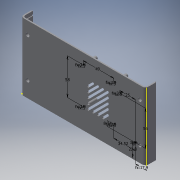
# Autodesk Inventor part: case-bottom
Saved by Autodesk Inventor 2017 (Build 210142000, 142)
## iProperties
Created: 2020-10-01
Part Number: case-bottom
Material: Generic
Document SubType Name: Modeling
Designer: jferner
Density: 1 g/cm^3
Appearance: Default
caseBottomDepth: 108.000 mm
caseBottomHeight: 17.000 mm
caseBottomWidth: 200.000 mm
thickness: 2.000 mm
fillet: 5.000 mm
frontBackOffset: -5.000 mm
filletInner: 3.000 mm
filletMid: 4.000 mm
lipHeight: 1.000 mm
offsetFromSideOfCase: 20.000 mm
caseJoinSpacingFrontBack: 63.000 mm
caseJoinSpacingLeftRight: 180.000 mm
caseJoinOffsetFromSide: 9.000 mm
caseJoinOffsetFromBack: 25.000 mm
caseJoinDiameter: 8.000 mm
holeDiameter: 3.400 mm
Author: jferner
Autodesk Inventor part; units mm, degrees
ref_plane "YZ Plane" through (0, 0, 0) normal (1, 0, 0) x (0, 1, 0)
ref_plane "XZ Plane" through (0, 0, 0) normal (0, 1, 0) x (-1, 0, 0)
ref_plane "XY Plane" through (0, 0, 0) normal (0, 0, 1) x (1, 0, 0)
sketch "Sketch1" plane through (0, 0, 0) normal (0, 0, 1) x (1, 0, 0)
  line L0 (0, 17) -> (0, 5)
  line L1 (5, 0) -> (195, 0)
  line L2 (200, 5) -> (200, 17)
  arc A0 (0, 5) -> (5, 0) centre (5, 5) ccw
  arc A1 (195, 0) -> (200, 5) centre (195, 5) ccw
  line L3 (2, 17) -> (2, 5)
  arc A2 (2, 5) -> (5, 2) centre (5, 5) ccw
  line L4 (5, 2) -> (195, 2)
  arc A3 (195, 2) -> (198, 5) centre (195, 5) ccw
  line L5 (198, 5) -> (198, 17)
  line L6 (0, 17) -> (2, 17)
  line L7 (198, 17) -> (200, 17)
  point P0 (0, 0)
  dimension "fillet" = 5
  dimension "thickness" = 2
  dimension "caseBottomWidth" = 200
  dimension "caseBottomHeight" = 17
  constraints: 16 end point, 8 point on circle, 4 centre point, 4 perpendicular, 4 tangent, 2 collinear, 2 point on line, 1 equal radius, 1 horizontal, 1 vertical, 4 other
  measures "fillet" radius of A0
  measures "thickness" distance between parallel lines of L0 L3
  measures "caseBottomWidth" distance between parallel lines of L2 L0
  measures "caseBottomHeight" distance between parallel lines of L6 L1
extrude "Extrusion1" add sketch "Sketch1" along normal blind 108
ref_plane "Work Plane1" through (0, 0, 103) normal (0, 0, 1) x (1, 0, 0)
sketch "Sketch3" plane through (0, 0, 103) normal (0, 0, 1) x (1, 0, 0)
  line L0 (2, 17) -> (1, 17)
  line L1 (2, 17) -> (2, 5)
  line L2 (1, 17) -> (1, 5)
  line L3 (195, 2) -> (5, 2) projected
  line L4 (195, 2) -> (5, 2)
  line L5 (198, 17) -> (198, 5) projected
  line L6 (198, 17) -> (198, 5)
  line L7 (198, 17) -> (199, 17)
  line L8 (199, 17) -> (199, 5)
  line L9 (5, 1) -> (195, 1)
  arc A0 (2, 5) -> (5, 2) centre (5, 5) ccw
  arc A1 (195, 2) -> (198, 5) centre (195, 5) ccw
  arc A2 (1, 5) -> (5, 1) centre (5, 5) ccw
  arc A3 (195, 1) -> (199, 5) centre (195, 5) ccw
  point P0 (0, 0)
  dimension "d8" = 1
  dimension "d9" = 1
  dimension "d10" = 1
  dimension "filletInner" = 3
  dimension "filletMid" = 4
  constraints: 16 end point, 8 point on circle, 8 tangent, 4 centre point, 4 horizontal, 3 vertical, 2 equal radius, 1 collinear, 1 parallel
  measures "d8" distance of L0.start L0.end
  measures "d9" distance of L5.start L7.end
  measures "d10" distance between parallel lines of L9 L4
  measures "filletInner" radius of A0
  measures "filletMid" radius of A2
extrude "Extrusion2" cut sketch "Sketch3" against normal blind 2
ref_plane "Work Plane2" through (0, 0, 5) normal (0, 0, -1) x (-1, 0, 0)
sketch "Sketch5" plane through (0, 0, 5) normal (0, 0, -1) x (-1, 0, 0)
  line L0 (-200, 17) -> (-198, 17) projected
  line L1 (-198, 17) -> (-198, 5)
  line L2 (-199, 17) -> (-199, 5)
  line L3 (-2, 5) -> (-2, 17) projected
  line L4 (-2, 17) -> (-2, 5)
  line L5 (-2, 17) -> (0, 17) projected
  line L6 (-1, 17) -> (-1, 5)
  line L7 (-195, 2) -> (-5, 2)
  line L8 (-195, 1) -> (-5, 1)
  line L9 (-195, 2) -> (-5, 2) projected
  arc A0 (-198, 5) -> (-195, 2) centre (-195, 5) ccw
  arc A1 (-5, 2) -> (-2, 5) centre (-5, 5) ccw
  arc A2 (-199, 5) -> (-195, 1) centre (-195, 5) ccw
  arc A3 (-5, 1) -> (-1, 5) centre (-5, 5) ccw
  point P0 (0, 0)
  dimension "d21" = 1
  dimension "d22" = 3
  dimension "d23" = 4
  constraints: 12 end point, 8 point on circle, 8 tangent, 4 centre point, 4 vertical, 2 equal radius, 2 horizontal, 2 midpoint, 1 collinear
  measures "d21" distance between parallel lines of L7 L8
  measures "d22" radius of A0
  measures "d23" radius of A2
extrude "Extrusion4" cut sketch "Sketch5" against normal blind 2
sketch "Sketch6" plane through (0, 0, 0) normal (0, 0, -1) x (-1, 0, 0)
  line L0 (-199, 17) -> (-199, 5) projected
  line L1 (-200, 5) -> (-200, 17) projected
  line L2 (-199, 17) -> (-200, 17)
  line L3 (-200, 17) -> (-200, 16)
  line L4 (-200, 16) -> (-199, 16)
  line L5 (-199, 16) -> (-199, 17)
  line L6 (-1, 17) -> (-1, 5) projected
  line L7 (0, 17) -> (-1, 17)
  line L8 (-1, 17) -> (-1, 16)
  line L9 (-1, 16) -> (0, 16)
  line L10 (0, 16) -> (0, 17)
  line L11 (0, 17) -> (0, 5) projected
  line L12 (-2, 17) -> (0, 17) projected
  point P0 (0, 0)
  dimension "lipHeight" = 1
  constraints: 16 end point, 4 parallel, 3 collinear, 2 horizontal, 2 perpendicular, 2 point on line
  measures "lipHeight" distance between parallel lines of L2 L4
extrude "Extrusion5" cut sketch "Sketch6" against normal through all
sketch "Sketch7" plane through (5, 2, 0) normal (0, 1, 0) x (1, 0, 0)
  circle A0 centre (177.1, -22.8) radius 2.5
  circle A1 centre (177.1, -22.8) radius 1.7
  circle A2 centre (142.58, -30.94) radius 2.5
  circle A3 centre (142.58, -30.94) radius 1.7
  circle A4 centre (142.58, -88.94) radius 2.5
  circle A5 centre (142.58, -88.94) radius 1.7
  circle A6 centre (93.58, -88.94) radius 2.5
  circle A7 centre (93.58, -88.94) radius 1.7
  circle A8 centre (93.58, -30.94) radius 2.5
  circle A9 centre (93.58, -30.94) radius 1.7
  circle A10 centre (152.1, -78.8) radius 2.5
  circle A11 centre (152.1, -78.8) radius 1.7
  line L0 (190, 0) -> (0, 0) projected
  line L1 (195, 0) -> (195, -108) projected
  point P0 (-5, 0)
  dimension "holeSupportDiameter" = 5
  dimension "holeDiameter" = 3.4
  dimension "d31" = 5
  dimension "d32" = 3.4
  dimension "d33" = 5
  dimension "d34" = 3.4
  dimension "d35" = 5
  dimension "d36" = 3.4
  dimension "d37" = 5
  dimension "d38" = 3.4
  dimension "d39" = 58
  dimension "d40" = 49
  dimension "d43" = 5
  dimension "d44" = 3.4
  dimension "d45" = 25
  dimension "d46" = 56
  dimension "d59" = 22.8
  dimension "d60" = 17.9
  dimension "d61" = 34.52
  dimension "d62" = 8.14
  constraints: 12 centre point, 6 coincident, 2 horizontal alignment, 2 vertical alignment
  measures "holeSupportDiameter" diameter of A0
  measures "holeDiameter" diameter of A1
  measures "d31" diameter of A2
  measures "d32" diameter of A3
  measures "d33" diameter of A4
  measures "d34" diameter of A5
  measures "d35" diameter of A6
  measures "d36" diameter of A7
  measures "d37" diameter of A8
  measures "d38" diameter of A9
  measures "d39" distance of A6.centre A8.centre
  measures "d40" distance of A6.centre A4.centre
  measures "d43" diameter of A10
  measures "d44" diameter of A11
  measures "d45" horizontal distance of A10.centre A0.centre
  measures "d46" vertical distance of A10.centre A0.centre
  measures "d59" distance from line of L0 A0.centre
  measures "d60" distance from line of L1 A0.centre
  measures "d61" horizontal distance of A0.centre A2.centre
  measures "d62" vertical distance of A2.centre A0.centre
extrude "Extrusion6" add sketch "Sketch7" along normal blind 22.5 contours A2 | A3 | A4 | A5 | A6 | A7 | A8 | A9
extrude "Extrusion7" add sketch "Sketch7" along normal blind 11.4 contours A0 | A1 | A10 | A11
sketch "Sketch8" plane through (182.1, 13.4, 22.8) normal (0, 1, 0) x (1, 0, 0)
  circle A0 centre (0, 0) radius 2.5 projected
  circle A1 centre (0, 0) radius 1.7
  circle A2 centre (-25, -56) radius 1.7
  circle A3 centre (-25, -56) radius 2.5 projected
  circle A4 centre (0, 0) radius 2.5 projected
  point P0 (-182.1, 22.8)
  point P1 (2.2499, -0.0186)
  point P2 (2.2499, 0.0186)
  dimension "d49" = 3.4
  dimension "d50" = 3.4
  constraints: 2 centre point, 1 coincident, 1 concentric, 3 other
  measures "d49" diameter of A1
  measures "d50" diameter of A2
extrude "Extrusion8" cut sketch "Sketch8" against normal blind 8 contours A1 | A2
sketch "Sketch9" plane through (147.58, 24.5, 30.94) normal (0, 1, 0) x (1, 0, 0)
  circle A0 centre (0, -58) radius 1.7
  circle A1 centre (0, 0) radius 1.7
  circle A2 centre (-49, 0) radius 1.7
  circle A3 centre (-49, -58) radius 2.5 projected
  circle A4 centre (-49, -58) radius 1.7
  circle A5 centre (0, -58) radius 2.5 projected
  circle A6 centre (0, 0) radius 2.5 projected
  circle A7 centre (-49, 0) radius 2.5 projected
  point P0 (-147.58, 30.94)
  dimension "d53" = 3.4
  dimension "d54" = 3.4
  dimension "d55" = 3.4
  dimension "d56" = 3.4
  constraints: 4 centre point, 3 concentric, 1 coincident
  measures "d53" diameter of A0
  measures "d54" diameter of A4
  measures "d55" diameter of A1
  measures "d56" diameter of A2
extrude "Extrusion9" cut sketch "Sketch9" against normal blind 8 contours A0 | A1 | A2 | A4
sketch "Sketch11" plane through (5, 0, 0) normal (0, -1, 0) x (1, 0, 0)
  line L0 (195, 0) -> (195, 108) projected
  line L1 (0, 108) -> (190, 108) projected
  line L2 (128.0253, 31.8538) -> (136.0525, 39.9311)
  line L3 (125.9203, 33.9457) -> (133.9475, 42.023)
  line L4 (136.0525, 48.0949) -> (119.9122, 31.8538)
  line L5 (117.8072, 33.9457) -> (133.9475, 50.1868)
  line L6 (112.1534, 31.8538) -> (136.0525, 55.9021)
  line L7 (133.9475, 57.9941) -> (110.0484, 33.9457)
  line L8 (104.1531, 31.8538) -> (136.0525, 63.9524)
  line L9 (133.9475, 66.0443) -> (102.0482, 33.9457)
  line L10 (104.1531, 39.8538) -> (136.0525, 71.9524)
  line L11 (133.9475, 74.0443) -> (102.0482, 41.9457)
  line L12 (104.1531, 47.8538) -> (128.1022, 71.9524)
  line L13 (125.9972, 74.0443) -> (102.0482, 49.9457)
  line L14 (104.1531, 55.8538) -> (120.1518, 71.9524)
  line L15 (118.0468, 74.0443) -> (102.0482, 57.9457)
  line L16 (104.1531, 63.8538) -> (112.2015, 71.9524)
  line L17 (110.0965, 74.0443) -> (102.0482, 65.9457)
  arc A0 (125.9203, 33.9457) -> (128.0253, 31.8538) centre (126.9728, 32.8997) ccw
  arc A1 (136.0525, 39.9311) -> (133.9475, 42.023) centre (135, 40.9771) ccw
  arc A2 (136.0525, 48.0949) -> (133.9475, 50.1868) centre (135, 49.1409) ccw
  arc A3 (136.0525, 55.9021) -> (133.9475, 57.9941) centre (135, 56.9481) ccw
  arc A4 (136.0525, 63.9524) -> (133.9475, 66.0443) centre (135, 64.9983) ccw
  arc A5 (136.0525, 71.9524) -> (133.9475, 74.0443) centre (135, 72.9983) ccw
  arc A6 (128.1022, 71.9524) -> (125.9972, 74.0443) centre (127.0497, 72.9983) ccw
  arc A7 (120.1518, 71.9524) -> (118.0468, 74.0443) centre (119.0993, 72.9983) ccw
  arc A8 (112.2015, 71.9524) -> (110.0965, 74.0443) centre (111.149, 72.9983) ccw
  arc A9 (102.0482, 65.9457) -> (104.1531, 63.8538) centre (103.1007, 64.8997) ccw
  arc A10 (102.0482, 57.9457) -> (104.1531, 55.8538) centre (103.1007, 56.8997) ccw
  arc A11 (102.0482, 49.9457) -> (104.1531, 47.8538) centre (103.1007, 48.8997) ccw
  arc A12 (102.0482, 41.9457) -> (104.1531, 39.8538) centre (103.1007, 40.8997) ccw
  arc A13 (102.0482, 33.9457) -> (104.1531, 31.8538) centre (103.1007, 32.8997) ccw
  arc A14 (110.0484, 33.9457) -> (112.1534, 31.8538) centre (111.1009, 32.8997) ccw
  arc A15 (117.8072, 33.9457) -> (119.9122, 31.8538) centre (118.8597, 32.8997) ccw
  point P0 (-5, 0)
  dimension "d162" = 60
  dimension "d163" = 67.0229
  dimension "d164" = 44.822
  dimension "d165" = 1.4838
  dimension "d166" = 11.3877
  dimension "d167" = 2.787
  dimension "d168" = 2.5356
  dimension "d169" = 2.7069
  dimension "d170" = 2.6715
  dimension "d171" = 2.6715
  dimension "d172" = 2.6715
  dimension "d173" = 2.6715
  dimension "d174" = 2.9677
  constraints: 32 end point, 32 point on circle, 29 tangent, 16 centre point, 15 parallel, 9 equal radius, 8 vertical alignment, 6 horizontal alignment
  measures "d162" distance from line of L0 A1.centre
  measures "d163" distance from line of L1 A1.centre
  measures "d164" angle of L0 L2
  measures "d165" radius of A0
  measures "d166" distance of A1.centre A0.centre
  measures "d167" distance between parallel lines of L4 L3
  measures "d168" distance between parallel lines of L6 L5
  measures "d169" distance between parallel lines of L8 L7
  measures "d170" distance between parallel lines of L10 L9
  measures "d171" distance between parallel lines of L12 L11
  measures "d172" distance between parallel lines of L14 L13
  measures "d173" distance between parallel lines of L16 L15
  measures "d174" distance between parallel lines of L2 L3
extrude "airHoles" cut sketch "Sketch11" against normal blind 4
sketch "Sketch12" plane through (5, 2, 101) normal (0, 1, 0) x (1, 0, 0)
  circle A0 centre (186, 76) radius 4
  line L0 (140.3029, -19.5933) -> (121.3678, -19.5933)
  line L1 (140.3029, -19.5933) -> (140.3029, -32.2167)
  circle A1 centre (186, 13) radius 4
  circle A2 centre (6, 76) radius 4
  circle A3 centre (6, 13) radius 4
  line L2 (195, 101) -> (195, -7) projected
  line L3 (190, 101) -> (0, 101) projected
  point P0 (-5, 101)
  dimension "caseJoinSpacingFrontBack" = 63
  dimension "caseJoinSpacingLeftRight" = 180
  dimension "caseJoinOffsetFromSide" = 9
  dimension "caseJoinOffsetFromBack" = 25
  dimension "caseJoinDiameter" = 8
  constraints: 4 centre point, 4 end point, 2 horizontal, 2 vertical, 6 other
  measures "caseJoinSpacingFrontBack" distance of A0.centre A1.centre
  measures "caseJoinSpacingLeftRight" distance of A0.centre A2.centre
  measures "caseJoinOffsetFromSide" distance from line of L2 A0.centre
  measures "caseJoinOffsetFromBack" distance from line of L3 A0.centre
  measures "caseJoinDiameter" diameter of A0
extrude "Extrusion12" add sketch "Sketch12" along normal blind 15
sketch "Sketch13" plane through (191, 17, 88) normal (0, 1, 0) x (1, 0, 0)
  circle A0 centre (0, 63) radius 4 projected
  circle A1 centre (0, 63) radius 1.7
  circle A2 centre (-180, 63) radius 4 projected
  circle A3 centre (-180, 63) radius 1.7
  circle A4 centre (-180, 0) radius 1.7
  circle A5 centre (-180, 0) radius 4 projected
  circle A6 centre (0, 0) radius 1.7
  circle A7 centre (0, 0) radius 4 projected
  point P0 (-191, 88)
  dimension "d154" = 3.4
  constraints: 4 centre point, 3 equal radius, 2 coincident, 2 concentric
  measures "d154" diameter of A1
extrude "Extrusion13" cut sketch "Sketch13" against normal through all contours A1 | A3 | A4 | A6
sketch "Sketch14" plane through (5, 0, 0) normal (0, -1, 0) x (1, 0, 0)
  circle A0 centre (186, 25) radius 3
  circle A1 centre (186, 25) radius 1.7 projected
  circle A2 centre (6, 88) radius 1.7 projected
  circle A3 centre (6, 88) radius 3
  circle A4 centre (186, 88) radius 1.7 projected
  circle A5 centre (186, 88) radius 3
  circle A6 centre (6, 25) radius 1.7 projected
  circle A7 centre (6, 25) radius 3
  point P0 (-5, 0)
  dimension "d157" = 6
  constraints: 4 centre point, 3 coincident, 3 equal radius, 1 concentric
  measures "d157" diameter of A0
extrude "Extrusion15" cut sketch "Sketch14" against normal blind 4
equation "\"d8\" = 0.5 * thickness"
equation "\"d9\" = 0.5 * thickness"
equation "\"d10\" = 0.5 * thickness"
equation "\"d13\" = thickness"
equation "\"d21\" = 0.5 * thickness"
equation "\"d22\" = filletInner"
equation "\"d23\" = filletMid"
equation "\"d24\" = thickness"
equation "\"d31\" = holeSupportDiameter"
equation "\"d32\" = holeDiameter"
equation "\"d33\" = holeSupportDiameter"
equation "\"d34\" = holeDiameter"
equation "\"d35\" = holeSupportDiameter"
equation "\"d36\" = holeDiameter"
equation "\"d37\" = holeSupportDiameter"
equation "\"d38\" = holeDiameter"
equation "\"d43\" = holeSupportDiameter"
equation "\"d44\" = holeDiameter"
equation "\"d49\" = holeDiameter"
equation "\"d50\" = holeDiameter"
equation "\"d53\" = holeDiameter"
equation "\"d54\" = holeDiameter"
equation "\"d55\" = holeDiameter"
equation "\"d56\" = holeDiameter"
equation "\"d57\" = holeDepth"
equation "\"d139\" = 2 * thickness"
equation "\"d152\" = caseBottomHeight - thickness"
equation "\"d154\" = holeDiameter"
equation "\"d15\" = frontBackOffset"
equation "\"offsetFromSideOfCase\" = 20"
equation "\"holeDepth\" = 8"
equation "\"frontBackOffset\" = -5"
body "Solid1" dims "d41" = 22.5 (computed from caseBottomHeight)
